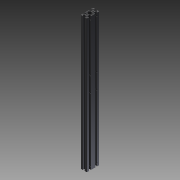
# Autodesk Inventor part: CAF5-2040-432-LCH-RCH-AH167-BH217
Saved by Autodesk Inventor 2011 SP1 (Build 150282100, 282)
## iProperties
Created: 2016-03-02
Part Number: CAF5-2040-432-LCH-RCH-AH167-BH217
Catalog Web Link: www.cadenas.de
Description: NFS5-2040, NFSB5-2040, HFS5-2040, HFSB5-2040, CAF5-2040, NFSF5-2040, HFSF5-2040-HFS5 Series Aluminum Extrusions 20,40 Square -2 Slots-
Vendor: MISUMI
Document SubType Name: Modeling
Designer: psAdmin
Manufacturer: MISUMI
Mass: 137.817 g
Surface Area: 1356.92 cm^2
Volume: 137.817 cm^3
Density: 1 g/cm^3
Category: PARTsolutions
Company: MISUMI
Title: CAF5-2040-432-LCH-RCH-AH167-BH217
Author: Cadenas PARTsolutions
Comments: HFS5 Series Aluminum Extrusions 20,40 Square -2 Slots-
PSOL_IDENT_0: {$CADENAS_DATA\23d-libs\misumi\metric\38_al_extrusions_blackets\5\hfs5_2040.prj},539 {VTYP=3D},{NB=C
PSOL_IDENT_1: AF5-2040-432-LCH-RCH-AH167-BH217},{LINA=CAF5-2040-432-LCH-RCH-AH167-BH217},{NN=NFS5-2040, NFSB5-2040
PSOL_IDENT_2: , HFS5-2040, HFSB5-2040, CAF5-2040, NFSF5-2040, HFSF5-2040},{DATE=17.07.2015 10:47:08},{GEOMDATE=28.
PSOL_IDENT_3: 10.2014 00:00:00},{VERSION=},{LINEID=130},{LINESUBID=-1},{WBVAR=L,ALT1,ALT2,ALT4,ALT5,CP5,DL5,DR5,AL
PSOL_IDENT_4: T6,ALT9,ALT10,ALT11,HP6,NHL6,DL6,NHR6,DR6,ALT7,ALT8,NH9,AH,BH,CH,DH,EH,NH10,AV,BV,CV,DV,EV,NH11,AP,B
PSOL_IDENT_5: P,CP,DP,EP,ALT12,ALT13,Z,NH12,XA,XB,XC,XD,XE,NH13,YA,YB,YC,YD,YE,ALT16,HP16,DL16,DR16,ALT17,HQ17,JLP
PSOL_IDENT_6: ,ALT18,HQ18,KLP,ALT20}  {NB=CAF5-2040-432-LCH-RCH-AH167-BH217},{LINA=CAF5-2040-432-LCH-RCH-AH167-BH2
PSOL_IDENT_7: 17},{KT=DUMMY},{PN=CAF5-2040-432-LCH-RCH-AH167-BH217},{TPS=CAF5-2040},{MAT=A6N01SS-T5 Aluminum Alloy
PSOL_IDENT_8: },{ST=Clear Coating (Anodize + Clear Coating)},{FRMW=20},{FRMH=40},{FRD=4.2},{L=432},{MASS=0.88},{SA=
PSOL_IDENT_9: 324},{LX=1.358x10^4},{LY=5.13x10^4},{ALT1=},{M1=0},{DPL1=0},{DPR1=0},{ALT1PN=},{ALT2=},{ALT2ALG= '','
PSOL_IDENT_10: w/o End Tapping (Heli-Coil Insert)','LHP','with LHP (Tapping on the Left (Heli-Coil Insert))','RHP','
PSOL_IDENT_11: with RHP (Tapping on the Right (Heli-Coil Insert))','HPW','with HPW (Tapping on Both Ends (Heli-Coil
PSOL_IDENT_12: Insert))' },{M2=0},{DP2=0},{ALT2PN=},{ALT4=},{ALT4ALG= '', 'w/o SC (High Precision Cut)', 'SC', 'wi
PSOL_IDENT_13: th SC (High Precision Cut)' },{ALT4PN=},{ALT5=},{ALT5ALG= '','w/o 45 Degree Cut','1','with 45 Degree
PSOL_IDENT_14: Cut' },{CP5=},{CP5ALG= '','N/A' },{DL5=},{DL5ALG= '','N/A' },{DR5=},{DR5ALG= '','N/A' },{FRMLALT5=0
PSOL_IDENT_15: },{FRMRALT5=0},{ALT5PN=},{ALT6=1},{ALT6ALG= '','w/o Fastening Location Wrench Access Hole Alteration
PSOL_IDENT_16: s','1','with Fastening Location Wrench Access Hole Alterations' },{ALT9=1},{ALT9ALG= '','w/o Locatio
PSOL_IDENT_17: n Specified Wrench Access Hole Alteratons (Horizontal)','1','with Location Specified Wrench Access H
PSOL_IDENT_18: ole Alteratons (Horizontal)' },{ALT10=},{ALT10ALG= '','w/o Location Specified Wrench Access Hole Alt
PSOL_IDENT_19: eratons (Vertical)','1','with Location Specified Wrench Access Hole Alteratons (Vertical)' },{ALT11=
PSOL_IDENT_20: },{ALT11ALG= '','w/o Location Specified Wrench Access Hole Alteratons (Crisscross)','1','with Locati
PSOL_IDENT_21: on Specified Wrench Access Hole Alteratons (Crisscross)' },{HP6=LR},{HP6ALG= 'L','Left','R','Right','
PSOL_IDENT_22: LR','Both Sides' },{NHL6=C},{NHL6ALG= 'C','C (Wrench Holes in Single Line)','W','W (Wrench Holes in
PSOL_IDENT_23: Two Lines)','E','E (Wrench Holes in Three Lines)' },{DL6=H},{DL6ALG= 'H','H (Horizontal)','V','V (Ve
PSOL_IDENT_24: rtical)','P','P (Crisscross)' },{NHR6=C},{NHR6ALG= 'C','C (Wrench Holes in Single Line)','W','W (Wre
PSOL_IDENT_25: nch Holes in Two Lines)','E','E (Wrench Holes in Three Lines)' },{DR6=H},{DR6ALG= 'H','H (Horizontal
PSOL_IDENT_26: )','V','V (Vertical)','P','P (Crisscross)' },{HL6=10},{HL6D=10},{HR6=10},{HR6D=10},{J6=20},{J6D=0},{
PSOL_IDENT_27: K6=20},{K6D=0},{DD6=7.35},{DD6ALG=7.35},{ALT7=},{ALT7ALG= '','w/o FL (Shifts The Wrench Hole on The
PSOL_IDENT_28: Left Side 3mm Toward The Left End)','FL','with FL (Shifts The Wrench Hole on The Left Side 3mm Towar
PSOL_IDENT_29: d The Left End)' },{ALT8=},{ALT8ALG= '','w/o FR (Shifts The Wrench Hole on The Right Side 3mm Toward
PSOL_IDENT_30: The Right End)','FR','with FR (Shifts The Wrench Hole on The Right Side 3mm Toward The Right End)'
PSOL_IDENT_31: },{ALT678PN=-LCH-RCH},{NH9=2},{NH9MAX=5},{NH9ALG=[1:5/1]},{AH=167.0},{AHMIN=7},{AHMAX=415.5},{AHALG=
PSOL_IDENT_32: [7:415.5/0.5]},{BH=217.0},{BHMIN=176.5},{BHMAX=425},{BHALG=[176.5:425/0.5]},{CH=0.0},{CHMIN=226.5},{
PSOL_IDENT_33: CHMAX=434.5},{CHALG=[0]},{DH=0.0},{DHMIN=9.5},{DHMAX=444},{DHALG=[0]},{EH=0.0},{EHMIN=9.5},{EHMAX=42
PSOL_IDENT_34: 5},{EHALG=[0]},{NH10=0},{NH10MAX=5},{NH10ALG=[0]},{AV=0.0},{AVMIN=7},{AVMAX=434.5},{AVALG=[0]},{BV=0
PSOL_IDENT_35: .0},{BVMIN=9.5},{BVMAX=444},{BVALG=[0]},{CV=0.0},{CVMIN=9.5},{CVMAX=453.5},{CVALG=[0]},{DV=0.0},{DVM
PSOL_IDENT_36: IN=9.5},{DVMAX=463},{DVALG=[0]},{EV=0.0},{EVMIN=9.5},{EVMAX=425},{EVALG=[0]},{NH11=0},{NH11MAX=5},{N
PSOL_IDENT_37: H11ALG=[0]},{AP=0.0},{APMIN=7},{APMAX=434.5},{APALG=[0]},{BP=0.0},{BPMIN=9.5},{BPMAX=444},{BPALG=[0]
PSOL_IDENT_38: },{CP=0.0},{CPMIN=9.5},{CPMAX=453.5},{CPALG=[0]},{DP=0.0},{DPMIN=9.5},{DPMAX=463},{DPALG=[0]},{EP=0.
PSOL_IDENT_39: 0},{EPMIN=9.5},{EPMAX=425},{EPALG=[0]},{ALT9PN=-AH167-BH217},{ALT10PN=},{ALT11PN=},{ALT91011PN=-AH16
PSOL_IDENT_40: 7-BH217},{ALT12=},{ALT12ALG= '','w/o Counterbore Hole in Specified Position (Vertical)','1','with Co
PSOL_IDENT_41: unterbore Hole in Specified Position (Vertical)' },{ALT13=},{ALT13ALG= '','w/o Counterbore Hole in S
PSOL_IDENT_42: pecified Position (Horizontal)','1','with Counterbore Hole in Specified Position (Horizontal)' },{Z=
PSOL_IDENT_43: },{ZALG= '','N/A' },{DD12=0.0},{DD112=0.0},{NH12=0},{NH12MAX=5},{NH12ALG=[0]},{XA=0.0},{XAMIN=7},{XA
PSOL_IDENT_44: MAX=427},{XAALG=[0]},{XB=0.0},{XBMIN=2},{XBMAX=429},{XBALG=[0]},{XC=0.0},{XCMIN=2},{XCMAX=431},{XCAL
PSOL_IDENT_45: G=[0]},{XD=0.0},{XDMIN=2},{XDMAX=433},{XDALG=[0]},{XE=0.0},{XEMIN=2},{XEMAX=425},{XEALG=[0]},{NH13=0
PSOL_IDENT_46: },{NH13MAX=5},{NH13ALG=[0]},{YA=0.0},{YAMIN=7},{YAMAX=427},{YAALG=[0]},{YB=0.0},{YBMIN=2},{YBMAX=429
PSOL_IDENT_47: },{YBALG=[0]},{YC=0.0},{YCMIN=2},{YCMAX=431},{YCALG=[0]},{YD=0.0},{YDMIN=2},{YDMAX=433},{YDALG=[0]},
PSOL_IDENT_48: {YE=0.0},{YEMIN=2},{YEMAX=425},{YEALG=[0]},{ALT12PN=},{ALT13PN=},{ALT1213PN=},{ALT16=},{ALT16ALG= ''
PSOL_IDENT_49: ,'w/o M Type Hole Alteration','1','with M Type Hole Alteration' },{HP16=},{HP16ALG= '','N/A' },{DL16=
PSOL_IDENT_50: },{DL16ALG= '','N/A' },{DR16=},{DR16ALG= '','N/A' },{H116=0},{D16=0.0},{ALT16PN=},{ALT17=},{ALT17ALG=
PSOL_IDENT_51: '','w/o L Type Hole Alteration (Top)','1','with L Type Hole Alteration (Top)' },{HQ17=0},{HQ17ALG=0
PSOL_IDENT_52: },{JLP=0},{JLPMIN=4.9},{JLPMAX=0},{JLPALG=[0]},{L17=0},{D17=0.0},{ALT18=},{ALT18ALG= '','w/o L Type
PSOL_IDENT_53: Hole Alteration (Bottom)','1','with L Type Hole Alteration (Bottom)' },{HQ18=0},{HQ18ALG=0},{KLP=0},
PSOL_IDENT_54: {KLPMIN=4.9},{KLPMAX=0},{KLPALG=[0]},{L18=0},{D18=0.0},{ALT1718PN=},{ALT20=},{ALT20PN=},{ERRORALT01=
PSOL_IDENT_55: OK},{ERRORALT02=OK},{ERRORALT05=OK},{ERRORALT06091=OK},{ERRORALT06092=OK},{ERRORALT06093=OK},{ERRORA
PSOL_IDENT_56: LT06094=OK},{ERRORALT06101=OK},{ERRORALT06102=OK},{ERRORALT06103=OK},{ERRORALT06104=OK},{ERRORALT061
PSOL_IDENT_57: 11=OK},{ERRORALT06112=OK},{ERRORALT06113=OK},{ERRORALT06114=OK},{ERRORALT06121=OK},{ERRORALT06122=OK
PSOL_IDENT_58: },{ERRORALT06123=OK},{ERRORALT06124=OK},{ERRORALT06131=OK},{ERRORALT06132=OK},{ERRORALT06133=OK},{ER
PSOL_IDENT_59: RORALT06134=OK},{ERRORALT0616=OK},{ERRORALT06171=OK},{ERRORALT06172=OK},{ERRORALT06173=OK},{ERRORALT
PSOL_IDENT_60: 06181=OK},{ERRORALT06182=OK},{ERRORALT06183=OK},{ERRORALT0911=OK},{ERRORALT0913=OK},{ERRORALT0916=OK
PSOL_IDENT_61: },{ERRORALT0917=OK},{ERRORALT0918=OK},{ERRORALT1011=OK},{ERRORALT1012=OK},{ERRORALT1016=OK},{ERRORAL
PSOL_IDENT_62: T1017=OK},{ERRORALT1018=OK},{ERRORALT1112=OK},{ERRORALT1113=OK},{ERRORALT1116=OK},{ERRORALT1117=OK},
PSOL_IDENT_63: {ERRORALT1118=OK},{ERRORALT1216=OK},{ERRORALT1217=OK},{ERRORALT1218=OK},{ERRORALT1316=OK},{ERRORALT1
PSOL_IDENT_64: 317=OK},{ERRORALT1318=OK},{ERRORALT1617=OK},{ERRORALT1618=OK},{ERRORPN=},{TFW=0}
NN: NFS5-2040, NFSB5-2040, HFS5-2040, HFSB5-2040, CAF5-2040, NFSF5-2040, HFSF5-2040
NT: HFS5 Series Aluminum Extrusions 20,40 Square -2 Slots-
NB: CAF5-2040-432-LCH-RCH-AH167-BH217
NBSYN: $PN.
LINA: CAF5-2040-432-LCH-RCH-AH167-BH217
PN: CAF5-2040-432-LCH-RCH-AH167-BH217
TPS: CAF5-2040
MAT: A6N01SS-T5 Aluminum Alloy
ST: Clear Coating (Anodize + Clear Coating)
L: 432
MASS: 0.88
SA: 324
LX: 1.358x10^4
LY: 5.13x10^4
ALT1: w/o End Tapping
M1: 0
DPL1: 0
DPR1: 0
ALT2: w/o End Tapping (Heli-Coil Insert)
M2: 0
DP2: 0
ALT4: w/o SC (High Precision Cut)
ALT5: w/o 45 Degree Cut
CP5: N/A
DL5: N/A
DR5: N/A
ALT6: with Fastening Location Wrench Access Hole Alterations
ALT9: with Location Specified Wrench Access Hole Alteratons (Horizontal)
ALT10: w/o Location Specified Wrench Access Hole Alteratons (Vertical)
ALT11: w/o Location Specified Wrench Access Hole Alteratons (Crisscross)
HP6: Both Sides
NHL6: C (Wrench Holes in Single Line)
DL6: H (Horizontal)
NHR6: C (Wrench Holes in Single Line)
DR6: H (Horizontal)
HL6D: 10
HR6D: 10
J6D: 0
K6D: 0
DD6: 7.35
ALT7: w/o FL (Shifts The Wrench Hole on The Left Side 3mm Toward The Left End)
ALT8: w/o FR (Shifts The Wrench Hole on The Right Side 3mm Toward The Right End)
NH9: 2
AH: 167.0
BH: 217.0
CH: 0.0
DH: 0.0
EH: 0.0
NH10: 0
AV: 0.0
BV: 0.0
CV: 0.0
DV: 0.0
EV: 0.0
NH11: 0
AP: 0.0
BP: 0.0
CP: 0.0
DP: 0.0
EP: 0.0
ALT12: w/o Counterbore Hole in Specified Position (Vertical)
ALT13: w/o Counterbore Hole in Specified Position (Horizontal)
Z: N/A
DD12: 0.0
DD112: 0.0
NH12: 0
XA: 0.0
XB: 0.0
XC: 0.0
XD: 0.0
XE: 0.0
NH13: 0
YA: 0.0
YB: 0.0
YC: 0.0
YD: 0.0
YE: 0.0
ALT16: w/o M Type Hole Alteration
HP16: N/A
DL16: N/A
DR16: N/A
H116: 0
D16: 0.0
ALT17: w/o L Type Hole Alteration (Top)
HQ17: 0
JLP: 0
D17: 0.0
ALT18: w/o L Type Hole Alteration (Bottom)
HQ18: 0
KLP: 0
D18: 0.0
ALT20: w/o CW (End Face C Chamfering)
SUPPLIER: MISUMI
ARTICLENO: CAF5-2040-432-LCH-RCH-AH167-BH217
BOMINFO: CAF5-2040-432-LCH-RCH-AH167-BH217
CREATOR: CADENAS GmbH
Autodesk Inventor part; units mm, degrees
sketch "Sketch_1" plane through (0, 0, 0) normal (0, 0, 1) x (1, 0, 0)
  arc A0 (-10, -19) -> (-9, -20) centre (-9, -19) ccw
  line L0 (-9, -20) -> (-3, -20)
  line L1 (-3, -20) -> (-3, -18)
  line L2 (-3, -18) -> (-6, -18)
  line L3 (-6, -18) -> (-6, -17.0607)
  line L4 (-6, -17.0607) -> (-2.9393, -14)
  line L5 (-2.9393, -14) -> (-0.5196, -14)
  line L6 (-0.5196, -14) -> (0, -13.7)
  line L7 (0, -13.7) -> (0.5196, -14)
  line L8 (0.5196, -14) -> (2.9393, -14)
  line L9 (2.9393, -14) -> (6, -17.0607)
  line L10 (6, -17.0607) -> (6, -18)
  line L11 (6, -18) -> (3, -18)
  line L12 (3, -18) -> (3, -20)
  line L13 (3, -20) -> (9, -20)
  arc A1 (9, -20) -> (10, -19) centre (9, -19) ccw
  line L14 (10, -19) -> (10, -13)
  line L15 (10, -13) -> (8, -13)
  line L16 (8, -13) -> (8, -16)
  line L17 (8, -16) -> (7.0607, -16)
  line L18 (7.0607, -16) -> (4, -12.9393)
  line L19 (4, -12.9393) -> (4, -10.5196)
  line L20 (4, -10.5196) -> (3.7, -10)
  line L21 (3.7, -10) -> (4, -9.4804)
  line L22 (4, -9.4804) -> (4, -7.0607)
  line L23 (4, -7.0607) -> (7.0607, -4)
  line L24 (7.0607, -4) -> (8, -4)
  line L25 (8, -4) -> (8, -7)
  line L26 (8, -7) -> (10, -7)
  line L27 (10, -7) -> (10, 7)
  line L28 (10, 7) -> (8, 7)
  line L29 (8, 7) -> (8, 4)
  line L30 (8, 4) -> (7.0607, 4)
  line L31 (7.0607, 4) -> (4, 7.0607)
  line L32 (4, 7.0607) -> (4, 9.4804)
  line L33 (4, 9.4804) -> (3.7, 10)
  line L34 (3.7, 10) -> (4, 10.5196)
  line L35 (4, 10.5196) -> (4, 12.9393)
  line L36 (4, 12.9393) -> (7.0607, 16)
  line L37 (7.0607, 16) -> (8, 16)
  line L38 (8, 16) -> (8, 13)
  line L39 (8, 13) -> (10, 13)
  line L40 (10, 13) -> (10, 19)
  arc A2 (10, 19) -> (9, 20) centre (9, 19) ccw
  line L41 (9, 20) -> (3, 20)
  line L42 (3, 20) -> (3, 18)
  line L43 (3, 18) -> (6, 18)
  line L44 (6, 18) -> (6, 17.0607)
  line L45 (6, 17.0607) -> (2.9393, 14)
  line L46 (2.9393, 14) -> (0.5196, 14)
  line L47 (0.5196, 14) -> (0, 13.7)
  line L48 (0, 13.7) -> (-0.5196, 14)
  line L49 (-0.5196, 14) -> (-2.9393, 14)
  line L50 (-2.9393, 14) -> (-6, 17.0607)
  line L51 (-6, 17.0607) -> (-6, 18)
  line L52 (-6, 18) -> (-3, 18)
  line L53 (-3, 18) -> (-3, 20)
  line L54 (-3, 20) -> (-9, 20)
  arc A3 (-9, 20) -> (-10, 19) centre (-9, 19) ccw
  line L55 (-10, 19) -> (-10, 13)
  line L56 (-10, 13) -> (-8, 13)
  line L57 (-8, 13) -> (-8, 16)
  line L58 (-8, 16) -> (-7.0607, 16)
  line L59 (-7.0607, 16) -> (-4, 12.9393)
  line L60 (-4, 12.9393) -> (-4, 10.5196)
  line L61 (-4, 10.5196) -> (-3.7, 10)
  line L62 (-3.7, 10) -> (-4, 9.4804)
  line L63 (-4, 9.4804) -> (-4, 7.0607)
  line L64 (-4, 7.0607) -> (-7.0607, 4)
  line L65 (-7.0607, 4) -> (-8, 4)
  line L66 (-8, 4) -> (-8, 7)
  line L67 (-8, 7) -> (-10, 7)
  line L68 (-10, 7) -> (-10, -7)
  line L69 (-10, -7) -> (-8, -7)
  line L70 (-8, -7) -> (-8, -4)
  line L71 (-8, -4) -> (-7.0607, -4)
  line L72 (-7.0607, -4) -> (-4, -7.0607)
  line L73 (-4, -7.0607) -> (-4, -9.4804)
  line L74 (-4, -9.4804) -> (-3.7, -10)
  line L75 (-3.7, -10) -> (-4, -10.5196)
  line L76 (-4, -10.5196) -> (-4, -12.9393)
  line L77 (-4, -12.9393) -> (-7.0607, -16)
  line L78 (-7.0607, -16) -> (-8, -16)
  line L79 (-8, -16) -> (-8, -13)
  line L80 (-8, -13) -> (-10, -13)
  line L81 (-10, -13) -> (-10, -19)
  arc A4 (-8, -1.7) -> (-7.7, -2) centre (-7.7, -1.7) ccw
  line L82 (-7.7, -2) -> (-7.0636, -2)
  arc A5 (-6.8515, -2.0879) -> (-7.0636, -2) centre (-7.0636, -2.3) ccw
  line L83 (-6.8515, -2.0879) -> (-2.9393, -6)
  line L84 (-2.9393, -6) -> (2.9393, -6)
  line L85 (2.9393, -6) -> (6.8515, -2.0879)
  arc A6 (7.0636, -2) -> (6.8515, -2.0879) centre (7.0636, -2.3) ccw
  line L86 (7.0636, -2) -> (7.7, -2)
  arc A7 (7.7, -2) -> (8, -1.7) centre (7.7, -1.7) ccw
  line L87 (8, -1.7) -> (8, 1.7)
  arc A8 (8, 1.7) -> (7.7, 2) centre (7.7, 1.7) ccw
  line L88 (7.7, 2) -> (7.0636, 2)
  arc A9 (6.8515, 2.0879) -> (7.0636, 2) centre (7.0636, 2.3) ccw
  line L89 (6.8515, 2.0879) -> (2.9393, 6)
  line L90 (2.9393, 6) -> (-2.9393, 6)
  line L91 (-2.9393, 6) -> (-6.8515, 2.0879)
  arc A10 (-7.0636, 2) -> (-6.8515, 2.0879) centre (-7.0636, 2.3) ccw
  line L92 (-7.0636, 2) -> (-7.7, 2)
  arc A11 (-7.7, 2) -> (-8, 1.7) centre (-7.7, 1.7) ccw
  line L93 (-8, 1.7) -> (-8, -1.7)
  constraints: 188 end point, 24 point on circle, 12 centre point
extrude "Extrusion1" add sketch "Sketch_1" against normal blind 432
sketch "Sketch2" plane through (0, 0, -432) normal (0, 0, -1) x (-1, 0, 0)
  point P0 (0, 10)
hole "Hole1" at (0, 10, -432) direction (0, 0, 1) diameter 4.2 depth 432
pattern_linear "Rectangular Pattern1" count 2 spacing 20 along (0, -1, 0) of "Hole1"
sketch "Sketch_13" plane through (0, 10, 0) normal (0, 1, 0) x (1, 0, 0)
  line L0 (10, 10) -> (-10, 10)
  line L1 (-10, 10) -> (-10, 13.675)
  line L2 (-10, 13.675) -> (10, 13.675)
  line L3 (10, 13.675) -> (10, 10)
  line L4 (10, 10) -> (-10, 10)
  constraints: 10 end point
revolve "Revolution1" cut sketch "Sketch_13" angle 360 about axis through (10, 10, -10) along (1, 0, 0)
sketch "_p_______11_Sketch_13_0" plane through (0, -10, 0) normal (0, 1, 0) x (1, 0, 0)
  line L0 (10, 10) -> (-10, 10)
  line L1 (-10, 10) -> (-10, 13.675)
  line L2 (-10, 13.675) -> (10, 13.675)
  line L3 (10, 13.675) -> (10, 10)
  line L4 (10, 10) -> (-10, 10)
  constraints: 10 end point
revolve "Revolution2" cut sketch "_p_______11_Sketch_13_0" angle 360 about axis through (10, -10, -10) along (1, 0, 0)
sketch "Sketch_16" plane through (0, 10, 0) normal (0, 1, 0) x (1, 0, 0)
  line L0 (10, 422) -> (-10, 422)
  line L1 (-10, 422) -> (-10, 425.675)
  line L2 (-10, 425.675) -> (10, 425.675)
  line L3 (10, 425.675) -> (10, 422)
  line L4 (10, 422) -> (-10, 422)
  constraints: 10 end point
revolve "Revolution3" cut sketch "Sketch_16" angle 360 about axis through (10, 10, -422) along (1, 0, 0)
sketch "_p_______14_Sketch_16_0" plane through (0, -10, 0) normal (0, 1, 0) x (1, 0, 0)
  line L0 (10, 422) -> (-10, 422)
  line L1 (-10, 422) -> (-10, 425.675)
  line L2 (-10, 425.675) -> (10, 425.675)
  line L3 (10, 425.675) -> (10, 422)
  line L4 (10, 422) -> (-10, 422)
  constraints: 10 end point
revolve "Revolution4" cut sketch "_p_______14_Sketch_16_0" angle 360 about axis through (10, -10, -422) along (1, 0, 0)
sketch "Sketch_62" plane through (0, 10, 0) normal (0, 1, 0) x (1, 0, 0)
  line L0 (10, 167) -> (-10, 167)
  line L1 (-10, 167) -> (-10, 170.675)
  line L2 (-10, 170.675) -> (10, 170.675)
  line L3 (10, 170.675) -> (10, 167)
  line L4 (10, 167) -> (-10, 167)
  constraints: 10 end point
revolve "Revolution5" cut sketch "Sketch_62" angle 360 about axis through (10, 10, -167) along (1, 0, 0)
sketch "_p_______17_Sketch_62_0" plane through (0, -10, 0) normal (0, 1, 0) x (1, 0, 0)
  line L0 (10, 167) -> (-10, 167)
  line L1 (-10, 167) -> (-10, 170.675)
  line L2 (-10, 170.675) -> (10, 170.675)
  line L3 (10, 170.675) -> (10, 167)
  line L4 (10, 167) -> (-10, 167)
  constraints: 10 end point
revolve "Revolution6" cut sketch "_p_______17_Sketch_62_0" angle 360 about axis through (10, -10, -167) along (1, 0, 0)
sketch "Sketch_25" plane through (0, 10, 0) normal (0, 1, 0) x (1, 0, 0)
  line L0 (10, 217) -> (-10, 217)
  line L1 (-10, 217) -> (-10, 220.675)
  line L2 (-10, 220.675) -> (10, 220.675)
  line L3 (10, 220.675) -> (10, 217)
  line L4 (10, 217) -> (-10, 217)
  constraints: 10 end point
revolve "Revolution7" cut sketch "Sketch_25" angle 360 about axis through (10, 10, -217) along (1, 0, 0)
sketch "_p_______18_Sketch_25_0" plane through (0, -10, 0) normal (0, 1, 0) x (1, 0, 0)
  line L0 (10, 217) -> (-10, 217)
  line L1 (-10, 217) -> (-10, 220.675)
  line L2 (-10, 220.675) -> (10, 220.675)
  line L3 (10, 220.675) -> (10, 217)
  line L4 (10, 217) -> (-10, 217)
  constraints: 10 end point
revolve "Revolution8" cut sketch "_p_______18_Sketch_25_0" angle 360 about axis through (10, -10, -217) along (1, 0, 0)
ref_plane "C1_XY" through (0, 0, 0) normal (0, 0, 1) x (1, 0, 0)
ref_plane "C1_YZ" through (0, 0, 0) normal (1, 0, 0) x (0, 1, 0)
ref_plane "C1_ZX" through (0, 0, 0) normal (0, 1, 0) x (0, 0, 1)
body "Solid1"
